Autodesk Fusion 360 part; units mm, degrees
(part 4 of 4)
sketch "Sketch19" plane through (0, 250, 0) normal (0, 1, 0) x (-1, 0, 0)
  line L0 (-99, 159) -> (-90, 159)
  line L1 (-90, 159) -> (-90, 150)
  line L2 (-90, 150) -> (-99, 150)
  line L3 (-99, 150) -> (-99, 159)
  line L4 (99, 159) -> (90, 159)
  line L5 (90, 159) -> (90, 150)
  line L6 (90, 150) -> (99, 150)
  line L7 (99, 150) -> (99, 159)
  dimension "d98" = 9
  dimension "d99" = 9
  dimension "d100" = 9
  dimension "d101" = 9
  constraint horizontal L0
  constraint vertical L1
  constraint horizontal L2
  constraint vertical L3
  constraint horizontal L4
  constraint vertical L5
  constraint horizontal L6
  constraint vertical L7
  measures "d98" distance of L0.start L0.end
  measures "d99" distance of L0.start L2.end
  measures "d100" distance of L4.start L4.end
  measures "d101" distance of L4.start L6.end
extrude "Extrude16" add sketch "Sketch19" along normal blind 20 separate body makes body 5 at (96, 256.6667, 159) makes body 6 at (-99, 256.6667, 153)
sketch "Sketch20" plane through (99, 0, 0) normal (1, 0, 0) x (0, 0, -1)
  line L0 (40, 37) -> (-150, 37)
  line L1 (-150, 37) -> (-150, 41.2426)
  line L2 (-150, 41.2426) -> (40, 41.2426)
  line L3 (40, 41.2426) -> (40, 37)
  line L4 (40, 51.2857) -> (-150, 51.2857)
  line L5 (-150, 51.2857) -> (-150, 55.5284)
  line L6 (-150, 55.5284) -> (40, 55.5284)
  line L7 (40, 55.5284) -> (40, 51.2857)
  line L8 (40, 65.5714) -> (-150, 65.5714)
  line L9 (-150, 65.5714) -> (-150, 69.8141)
  line L10 (-150, 69.8141) -> (40, 69.8141)
  line L11 (40, 69.8141) -> (40, 65.5714)
  line L12 (40, 79.8571) -> (-150, 79.8571)
  line L13 (-150, 79.8571) -> (-150, 84.0998)
  line L14 (-150, 84.0998) -> (40, 84.0998)
  line L15 (40, 84.0998) -> (40, 79.8571)
  line L16 (40, 94.1429) -> (-150, 94.1429)
  line L17 (-150, 94.1429) -> (-150, 98.3855)
  line L18 (-150, 98.3855) -> (40, 98.3855)
  line L19 (40, 98.3855) -> (40, 94.1429)
  line L20 (40, 108.4286) -> (-150, 108.4286)
  line L21 (-150, 108.4286) -> (-150, 112.6712)
  line L22 (-150, 112.6712) -> (40, 112.6712)
  line L23 (40, 112.6712) -> (40, 108.4286)
  line L24 (40, 122.7143) -> (-150, 122.7143)
  line L25 (-150, 122.7143) -> (-150, 126.9569)
  line L26 (-150, 126.9569) -> (40, 126.9569)
  line L27 (40, 126.9569) -> (40, 122.7143)
  line L28 (40, 137) -> (-150, 137)
  line L29 (-150, 137) -> (-150, 141.2426)
  line L30 (-150, 141.2426) -> (40, 141.2426)
  line L31 (40, 141.2426) -> (40, 137)
  line L32 (40, 151.2857) -> (-150, 151.2857)
  line L33 (-150, 151.2857) -> (-150, 155.5284)
  line L34 (-150, 155.5284) -> (40, 155.5284)
  line L35 (40, 155.5284) -> (40, 151.2857)
  line L36 (40, 165.5714) -> (-150, 165.5714)
  line L37 (-150, 165.5714) -> (-150, 169.8141)
  line L38 (-150, 169.8141) -> (40, 169.8141)
  line L39 (40, 169.8141) -> (40, 165.5714)
  line L40 (40, 179.8571) -> (-150, 179.8571)
  line L41 (-150, 179.8571) -> (-150, 184.0998)
  line L42 (-150, 184.0998) -> (40, 184.0998)
  line L43 (40, 184.0998) -> (40, 179.8571)
  line L44 (40, 194.1429) -> (-150, 194.1429)
  line L45 (-150, 194.1429) -> (-150, 198.3855)
  line L46 (-150, 198.3855) -> (40, 198.3855)
  line L47 (40, 198.3855) -> (40, 194.1429)
  line L48 (40, 208.4286) -> (-150, 208.4286)
  line L49 (-150, 208.4286) -> (-150, 212.6712)
  line L50 (-150, 212.6712) -> (40, 212.6712)
  line L51 (40, 212.6712) -> (40, 208.4286)
  line L52 (40, 222.7143) -> (-150, 222.7143)
  line L53 (-150, 222.7143) -> (-150, 226.9569)
  line L54 (-150, 226.9569) -> (40, 226.9569)
  line L55 (40, 226.9569) -> (40, 222.7143)
  line L56 (40, 241.2426) -> (40, 237)
  line L57 (40, 237) -> (-150, 237)
  line L58 (-150, 237) -> (-150, 241.2426)
  line L59 (-150, 241.2426) -> (40, 241.2426)
  line L60 (-159, 250) -> (-159, 18)
  line L61 (-159, 18) -> (49, 18)
  line L62 (49, 18) -> (49, 280)
  line L63 (49, 280) -> (40, 280)
  line L64 (40, 280) -> (40, 250)
  line L65 (40, 250) -> (-159, 250)
  line L66 (49, 280) -> (-159, 270)
  line L67 (-159, 270, 0) -> (-159, 270, -198)
  line L68 (-159, 270, -198) -> (49, 280, -198)
  line L69 (49, 280, -198) -> (49, 280, 0)
  point P0 (-159, 270)
  point P1 (-159, 270)
  point P2 (49, 280)
  constraint coincident P2 L62.end
  constraint coincident P1 P0
extrude "Extrude17" add sketch "Sketch20" along normal blind 5 contours L66 L67 L68 L69 in plane through (99, 277.004, 13.3175) normal (0, 0.998846, 0.048021) bodies 1 5 6
sketch "Sketch21" plane through (0, 0, 0) normal (0, 1, 0) x (1, 0, 0)
component "Component" placed x (1, 0, 0) y (0, 1, 0) z (0, 0, 1) at (-80, 0, 0)
